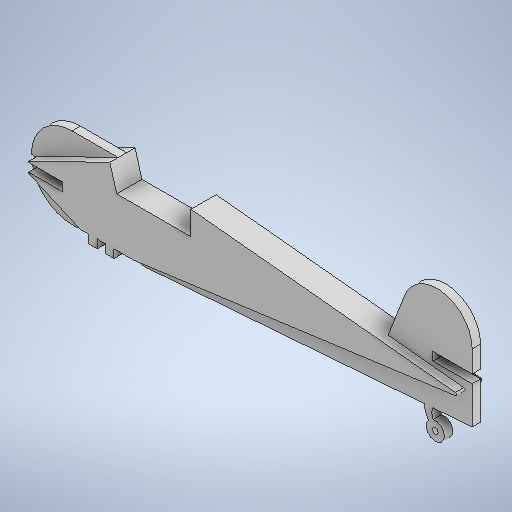
# Autodesk Inventor part: CORPO
Saved by Autodesk Inventor 2025.1 (Build 291241000, 241)
## iProperties
Created: 2024-10-26
Part Number: CORPO
Material: Genérico
Document SubType Name: Modeling
Designer: ambrosildo
Density: 1 g/cm^3
Appearance: Padrão
Author: ambrosildo
Autodesk Inventor part; units mm, degrees
ref_plane "YZ Plane" through (0, 0, 0) normal (1, 0, 0) x (0, 1, 0)
ref_plane "XZ Plane" through (0, 0, 0) normal (0, 1, 0) x (-1, 0, 0)
ref_plane "XY Plane" through (0, 0, 0) normal (0, 0, 1) x (1, 0, 0)
sketch "Esboço1" plane through (0, 0, 0) normal (0, 0, 1) x (1, 0, 0)
  line L0 (0, 0) -> (143, 0)
  line L1 (0, 14.5) -> (16.5, 14.5)
  line L2 (45.5, 14.5) -> (45.5, 6)
  line L3 (143, 0) -> (113, 0)
  line L4 (45.5, 14.5) -> (113, 7.75)
  arc A0 (143, 18.4741) -> (118.8287, 22.9497) centre (130.5, 18.4741) ccw
  line L5 (113, 7.75) -> (118.8287, 22.9497)
  line L6 (0, -14.5) -> (2, -14.5)
  line L7 (2, -14.5) -> (2, -11.5)
  line L8 (18.9914, 6) -> (45.5, 6)
  line L9 (16.5, 14.5) -> (18.9914, 6)
  line L10 (27, -14.5) -> (25, -14.5)
  line L11 (25, -14.5) -> (25, -11.5)
  line L12 (2, -11.5) -> (25, -11.5)
  line L13 (143, -5.6516) -> (129.0406, -6.7164)
  arc A1 (127.3817, -11.2647) -> (129.06, -10.2586) centre (129.8143, -13.4198) ccw
  circle A2 centre (129.8143, -13.4198) radius 1
  arc A3 (126.0492, -6.9446) -> (127.3817, -11.2647) centre (132.7451, -7.2449) ccw
  arc A4 (129.0406, -6.7164) -> (129.06, -10.2586) centre (132.2697, -8.4698) ccw
  line L14 (27, -14.5) -> (126.0492, -6.9446)
  line L15 (129.0406, -6.7164) -> (143, -5.6516)
  line L16 (-14.5, 0) -> (-0.5, 0)
  line L17 (-0.5, 0) -> (-0.5, -3)
  line L18 (-0.5, -3) -> (-14.1863, -3)
  arc A5 (0, 14.5) -> (-14.5, 0) centre (0, 0) ccw
  arc A6 (-14.1863, -3) -> (0, -14.5) centre (0, 0) ccw
  line L19 (113, 7.75) -> (124.9404, 6.556)
  line L20 (143, 10.75) -> (129, 10.75)
  line L21 (129, 10.75) -> (129, 7.75)
  line L22 (129, 7.75) -> (143, 7.75)
  line L23 (143, -5.6516) -> (143, 7.75)
  line L24 (143, 10.75) -> (143, 18.4741)
  dimension "d1" = 143
  dimension "d5" = 29
  dimension "d6" = 8.5
  dimension "d23" = 2
  dimension "d24" = 3
  dimension "d67" = 6.5
  dimension "d68" = 2
  dimension "d85" = 14
  dimension "d86" = 3
  dimension "d87" = 12
  dimension "d91" = 14
  constraints: 50 end point, 12 point on circle, 7 centre point, 5 perpendicular, 4 horizontal, 4 tangent, 2 coincident, 2 point on line, 2 vertical
  measures "d1" distance of L0.start L0.end
  measures "d5" distance of L1.end L2.start
  measures "d6" distance of L2.start L2.end
  measures "d23" distance of L6.start L6.end
  measures "d24" distance of L6.end L7.end
  measures "d67" diameter of A1
  measures "d68" diameter of A2
  measures "d85" distance of L16.start L16.end
  measures "d86" distance of L16.end L17.end
  measures "d87" distance of L4.end L19.end
  measures "d91" distance of L20.start L20.end
extrude "Extrusão1" add sketch "Esboço1" along normal blind 3
sketch "Esboço2" plane through (0, 0, 3) normal (0, 0, 1) x (1, 0, 0)
  line L0 (113, 7.75) -> (45.5, 14.5) projected
  line L1 (45.5, 14.5) -> (140.0285, 5.0471)
  arc A0 (140.0458, 4.0541) -> (140.0285, 5.0471) centre (139.9788, 4.5496) ccw
  line L2 (18.9914, 6) -> (16.5, 14.5) projected
  line L3 (25, -11.5) -> (140.0458, 4.0541)
  line L4 (45.5, 6) -> (18.9914, 6) projected
  line L5 (18.9914, 6) -> (45.5, 6)
  line L6 (45.5, 6) -> (45.5, 14.5)
  line L7 (9, -11.5) -> (9, -14.5)
  line L8 (9, -14.5) -> (12, -14.5)
  line L9 (12, -14.5) -> (12, -11.5)
  line L10 (6, -11.5) -> (9, -11.5)
  line L11 (18, -11.5) -> (18, -14.5)
  line L12 (18, -14.5) -> (15, -14.5)
  line L13 (15, -14.5) -> (15, -11.5)
  line L14 (12, -11.5) -> (15, -11.5)
  line L15 (18, -11.5) -> (25, -11.5)
  line L16 (-12.5, 0) -> (-12.5, 0.25)
  arc A1 (-12.3593, 0.4749) -> (-12.5, 0.25) centre (-12.25, 0.25) ccw
  line L17 (16.5, 14.5) -> (-12.3593, 0.4749)
  line L18 (-12.5, -3) -> (-12.5, -3.25)
  arc A2 (-12.5, -3.25) -> (-12.3501, -3.4791) centre (-12.25, -3.25) ccw
  line L19 (6, -11.5) -> (-12.3501, -3.4791)
  line L20 (-12.5, 0) -> (-0.5, 0)
  line L21 (-0.5, 0) -> (-0.5, -3)
  line L22 (-0.5, -3) -> (-12.5, -3)
  point P0 (0, 0)
  point P1 (113, 7.75)
  dimension "d22" = 95
  dimension "d45" = 3
  dimension "d46" = 3
  dimension "d48" = 3
  dimension "d49" = 3
  dimension "d60" = 3
  dimension "d82" = 12
  constraints: 40 end point, 6 perpendicular, 6 point on circle, 3 centre point, 3 tangent, 2 collinear, 2 horizontal, 2 vertical, 1 parallel
  measures "d22" distance of L0.end L1.end
  measures "d45" distance of L7.start L7.end
  measures "d46" distance of L7.end L8.end
  measures "d48" distance of L11.end L12.end
  measures "d49" distance of L11.start L11.end
  measures "d60" distance of L16.start L18.start
  measures "d82" distance of L16.start L20.end
extrude "Extrusão2" add sketch "Esboço2" along normal blind 3
sketch "Esboço3" plane through (0, 0, 0) normal (0, 0, -1) x (-1, 0, 0)
  arc A0 (-140.0285, 5.0471) -> (-140.0458, 4.0541) centre (-139.9788, 4.5496) ccw projected
  arc A1 (-140.0285, 5.0471) -> (-140.0458, 4.0541) centre (-139.9788, 4.5496) ccw
  line L0 (-25, -11.5) -> (-140.0458, 4.0541)
  line L1 (-45.5, 14.5) -> (-45.5, 6) projected
  line L2 (-45.5, 14.5) -> (-45.5, 6)
  line L3 (-45.5, 6) -> (-18.9914, 6)
  line L4 (-25, -11.5) -> (-18, -11.5)
  line L5 (-18.9914, 6) -> (-16.5, 14.5)
  arc A2 (12.5, 0.25) -> (12.3593, 0.4749) centre (12.25, 0.25) ccw projected
  arc A3 (12.5, 0.25) -> (12.3593, 0.4749) centre (12.25, 0.25) ccw
  arc A4 (12.3501, -3.4791) -> (12.5, -3.25) centre (12.25, -3.25) ccw projected
  arc A5 (12.3501, -3.4791) -> (12.5, -3.25) centre (12.25, -3.25) ccw
  line L6 (-15, -14.5) -> (-18, -14.5) projected
  line L7 (-18, -11.5) -> (-18, -14.5)
  line L8 (-18, -14.5) -> (-15, -14.5)
  line L9 (-15, -14.5) -> (-15, -11.5)
  line L10 (-12, -14.5) -> (-12, -11.5) projected
  line L11 (-15, -11.5) -> (-12, -11.5)
  line L12 (-12, -11.5) -> (-12, -14.5)
  line L13 (-9, -11.5) -> (-9, -14.5) projected
  line L14 (-12, -14.5) -> (-9, -14.5)
  line L15 (-9, -14.5) -> (-9, -11.5)
  line L16 (12.3501, -3.4791) -> (-6, -11.5) projected
  line L17 (-9, -11.5) -> (-6, -11.5)
  line L18 (-6, -11.5) -> (12.3501, -3.4791)
  line L19 (-16.5, 14.5) -> (12.3593, 0.4749) projected
  line L20 (-16.5, 14.5) -> (12.3593, 0.4749)
  line L21 (-140.0285, 5.0471) -> (-45.5, 14.5) projected
  line L22 (-45.5, 14.5) -> (-140.0285, 5.0471)
  line L23 (12.5, -3.25) -> (12.5, -3)
  line L24 (12.5, 0) -> (12.5, 0.25)
  line L25 (12.5, 0) -> (0.5, 0)
  line L26 (0.5, 0) -> (0.5, -3)
  line L27 (0.5, -3) -> (12.5, -3)
  point P0 (12.3501, -3.4791)
  point P1 (12.3593, 0.4749)
  point P2 (12.3593, 0.4749)
  point P3 (12.5, 0.25)
  point P4 (12.5, -3.25)
  point P5 (12.3501, -3.4791)
  constraints: 43 end point, 13 tangent, 7 collinear, 7 perpendicular, 6 point on circle, 3 centre point, 3 coincident, 2 horizontal
extrude "Extrusão3" add sketch "Esboço3" along normal blind 3
